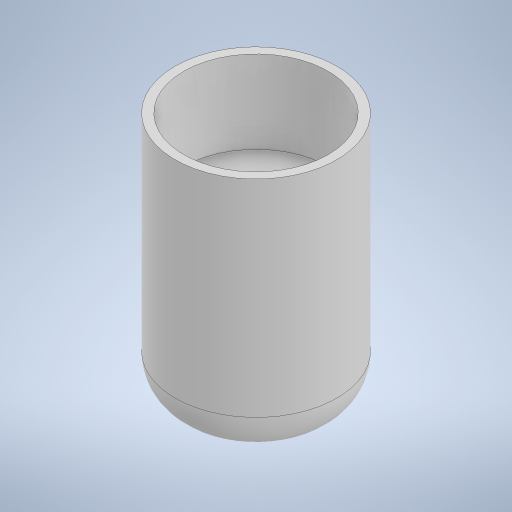
# Autodesk Inventor part: Casquillo
Saved by Autodesk Inventor 2024 (Build 280153000, 153)
## iProperties
Created: 2023-11-25
Part Number: Casquillo
Material: Genérico
Document SubType Name: Modeling
Designer: sergi
Density: 1 g/cm^3
Appearance: Valor por defecto
Author: sergi
Autodesk Inventor part; units mm, degrees
ref_plane "YZ Plane" through (0, 0, 0) normal (1, 0, 0) x (0, 1, 0)
ref_plane "XZ Plane" through (0, 0, 0) normal (0, 1, 0) x (-1, 0, 0)
ref_plane "XY Plane" through (0, 0, 0) normal (0, 0, 1) x (1, 0, 0)
sketch "Boceto1" plane through (0, 0, 0) normal (0, 1, 0) x (-1, 0, 0)
  circle A0 centre (0, 0) radius 19.6
  dimension "d0" = 39.2
  constraints: 1 centre point, 1 coincident
  measures "d0" diameter of A0
extrude "Extrusión1" add sketch "Boceto1" along normal blind 60
sketch "Boceto2" plane through (0, 60, 0) normal (0, 1, 0) x (1, 0, 0)
  circle A0 centre (0, 0) radius 19.6 projected
  constraints: 1 coincident
hole "Agujero1" at (0, 60, 0) direction (0, -1, 0) diameter 35 depth 20 tip angle 118
sketch "Boceto3" plane through (0, 0, 0) normal (0, -1, 0) x (1, 0, 0)
  circle A0 centre (0, 0) radius 19.6 projected
  constraints: 1 coincident
hole "Agujero2" at (0, 0, 0) direction (0, 1, 0) diameter 10 depth 20 tip angle 118
thread "Rosca1" size "M10x1.5" class "6H" standard "ANSI Metric M Profile" full length
fillet "Empalme1" radius 10 1 edges at (19.6, 0, 0)
